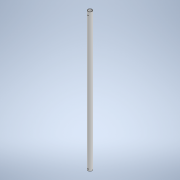
# Autodesk Inventor part: airfoil
Saved by Autodesk Inventor 2022 (Build 260153000, 153)
## iProperties
Created: 2021-03-06
Part Number: airfoil
Material: Generic
Document SubType Name: Modeling
Designer: Ferdinand Hubbard
Density: 1 g/cm^3
Appearance: Default
Author: Ferdinand Hubbard
Autodesk Inventor part; units mm, degrees
ref_plane "YZ Plane" through (0, 0, 0) normal (1, 0, 0) x (0, 1, 0)
ref_plane "XZ Plane" through (0, 0, 0) normal (0, 1, 0) x (-1, 0, 0)
ref_plane "XY Plane" through (0, 0, 0) normal (0, 0, 1) x (1, 0, 0)
sketch "Sketch2" plane through (0, 0, 0) normal (0, 1, 0) x (-1, 0, 0)
  circle A0 centre (0, 0) radius 7.5
  circle A1 centre (0, 0) radius 6.5
  dimension "d91" = 15
  dimension "d92" = 13
  constraints: 2 centre point, 2 coincident
  measures "d91" diameter of A0
  measures "d92" diameter of A1
extrude "Extrusion5" add sketch "Sketch2" along normal blind 500
sketch "Sketch3" plane through (0, 0, 0) normal (0, 0, 1) x (1, 0, 0)
  line L0 (0, 0) -> (0, 6)
  circle A0 centre (0, 6) radius 1.5
  line L1 (7.5, 500) -> (-7.5, 500) projected
  line L2 (0, 500) -> (0, 488)
  circle A1 centre (0, 488) radius 1.5
  dimension "d95" = 6
  dimension "d96" = 3
  dimension "d101" = 12
  dimension "d102" = 3
  constraints: 4 end point, 2 centre point, 2 coincident, 2 vertical, 1 midpoint
  measures "d95" distance of L0.start L0.end
  measures "d96" diameter of A0
  measures "d101" distance of L2.start L2.end
  measures "d102" diameter of A1
extrude "Extrusion6" cut sketch "Sketch3" along normal blind 20 and the other way blind 10
body "Solid5"
